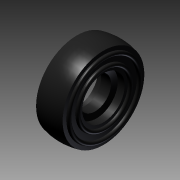
# Autodesk Inventor part: 3139
Saved by Autodesk Inventor 2011 SP1 (Build 150282100, 282)
## iProperties
Created: 2011-09-28
Part Number: 3139
Cost Center: 0 kg
Material: Steel
Document SubType Name: Modeling
Designer: PMe
Authority: 0 mm^3
Stock Number: =<Filenr>_<Document number>
Density: 7.85 g/cm^3
Company: Allseas Engineering BV
Subject: =<Title><TITLE 1_2> <TITLE 2_2>
Author: PMe
Act. Code: DW000
SaveDate: 2011-07-28
SaveTime: 18:32
FileName: Standard
TotalMass: 0 kg
TotalVolume: 0 mm^3
Autodesk Inventor part; units mm, degrees
ref_plane "YZ Plane" through (0, 0, 0) normal (1, 0, 0) x (0, 1, 0)
ref_plane "XZ Plane" through (0, 0, 0) normal (0, 1, 0) x (-1, 0, 0)
ref_plane "XY Plane" through (0, 0, 0) normal (0, 0, 1) x (1, 0, 0)
sketch "Sketch1" plane through (0, 0, 0) normal (0, 0, 1) x (1, 0, 0)
  arc A0 (-2.5, -7.6825) -> (2.5, -7.6825) centre (0, 2) ccw
  line L0 (-2.5, -7.6825) -> (-2.5, -6.9825)
  line L1 (-2.5, -6.9825) -> (-3, -6.9825)
  line L2 (-3, -6.9825) -> (-3, -6.2825)
  line L3 (-3, -6.2825) -> (-2.5, -6.2825)
  line L4 (-2.5, -6.2825) -> (-2.5, -5.2825)
  line L5 (-2.5, -5.2825) -> (-3, -5.2825)
  line L6 (-3, -5.2825) -> (-3, -4.5825)
  line L7 (-3, -4.5825) -> (-2.5, -4.5825)
  line L8 (-2.5, -4.5825) -> (-2.5, -4)
  line L9 (-2.5, -4) -> (-1.2, -4)
  line L10 (-1.2, -4) -> (-0.9333, -3)
  line L11 (-0.9333, -3) -> (0.9333, -3)
  line L12 (0.9333, -3) -> (1.2, -4)
  line L13 (1.2, -4) -> (2.5, -4)
  line L14 (2.5, -4) -> (2.5, -4.5825)
  line L15 (2.5, -4.5825) -> (3, -4.5825)
  line L16 (3, -4.5825) -> (3, -5.2825)
  line L17 (3, -5.2825) -> (2.5, -5.2825)
  line L18 (2.5, -5.2825) -> (2.5, -6.2825)
  line L19 (2.5, -6.2825) -> (3, -6.2825)
  line L20 (3, -6.2825) -> (3, -6.9825)
  line L21 (3, -6.9825) -> (2.5, -6.9825)
  line L22 (2.5, -6.9825) -> (2.5, -7.6825)
  line L23 (-6.3827, 0) -> (6.3827, 0)
  line L24 (0, 0) -> (0, -8) construction
  line L25 (-0.9333, -3) -> (-0.8, -2.5) construction
  line L26 (-0.8, -2.5) -> (0.8, -2.5) construction
  line L27 (0.8, -2.5) -> (0.9333, -3) construction
  point P0 (0, -3)
  dimension "d0" = 5
  dimension "d1" = 6
  dimension "d2" = 6
  dimension "d3" = 0.7
  dimension "d4" = 16
  dimension "d5" = 1
  dimension "d6" = 10
  dimension "d7" = 2.4
  dimension "d8" = 8
  dimension "d9" = 1.5
  dimension "d10" = 1.6
  constraints: 56 end point, 13 perpendicular, 12 equal length, 7 parallel, 6 vertical alignment, 4 collinear, 3 point on circle, 2 midpoint, 1 centre point, 1 coincident, 1 vertical
  measures "d0" distance between parallel lines of L22 L0
  measures "d1" diameter of L11 L23
  measures "d2" distance between parallel lines of L20 L2
  measures "d3" distance of L19.end L20.end
  measures "d4" diameter of L24.end L23
  measures "d5" distance of L17.end L18.end
  measures "d6" radius of A0
  measures "d7" distance of L12.end L9.end
  measures "d8" diameter of L9 L23
  measures "d9" distance between parallel lines of L26 L13
  measures "d10" distance of L25.end L26.end
revolve "Revolution1" add sketch "Sketch1" angle 360 about axis through (-6.3827, 0, 0) along (1, 0, 0)
fillet "Fillet1" radius 0.35 8 edges at (3, 6.9825, 0) (3, 6.2825, 0) (3, 5.2825, 0) (3, 4.5825, 0) (-3, 6.2825, 0) (-3, 4.5825, 0) (-3, 6.9825, 0) (-3, 5.2825, 0)
body "Solid1"
